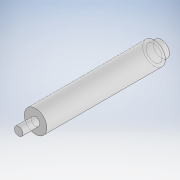
# Autodesk Inventor part: Pok X-Carriage Top Support
Saved by Autodesk Inventor 2018.2 (Build 222227000, 227)
## iProperties
Created: 2018-02-08
Part Number: Pok X-Carriage Top Support
Material: ABS Plastic
Document SubType Name: Modeling
Designer: Moochster
Density: 1.06 g/cm^3
Appearance: Smooth - White
Author: Moochster
Autodesk Inventor part; units mm, degrees
ref_plane "YZ Plane" through (0, 0, 0) normal (1, 0, 0) x (0, 1, 0)
ref_plane "XZ Plane" through (0, 0, 0) normal (0, 1, 0) x (-1, 0, 0)
ref_plane "XY Plane" through (0, 0, 0) normal (0, 0, 1) x (1, 0, 0)
sketch "Sketch1" plane through (0, 0, 0) normal (0, 0, 1) x (1, 0, 0)
  line L0 (0, 0) -> (0, 50.5)
  line L1 (0, 50.5) -> (2.85, 50.5)
  line L2 (2.85, 50.5) -> (2.85, 47.9)
  line L3 (2.85, 47.9) -> (4, 47.9)
  line L4 (4, 47.9) -> (4, 6)
  line L5 (4, 6) -> (1.5, 6)
  line L6 (1.5, 6) -> (1.5, 0)
  line L7 (1.5, 0) -> (0, 0)
  dimension "d0" = 3
  dimension "d1" = 6
  dimension "d2" = 50.5
  dimension "d3" = 5.7
  dimension "d4" = 8
  dimension "d5" = 2.6
  constraints: 16 end point, 6 perpendicular, 1 horizontal, 1 vertical
  measures "d0" diameter of L6 L0
  measures "d1" distance of L5.end L6.end
  measures "d2" distance of L0.start L0.end
  measures "d3" diameter of L2 L0
  measures "d4" diameter of L4 L0
  measures "d5" distance of L1.end L2.end
revolve "Revolution1" add sketch "Sketch1" angle 360 about axis through (0, 0, 0) along (0, 1, 0)
body "Solid1"
